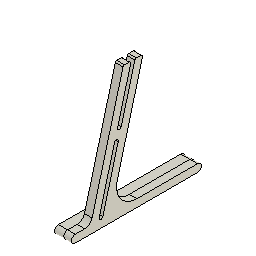
LCA 2021 Badge Stand v3 (Autodesk Fusion 360 design; units mm, degrees)
Autodesk Fusion 360 part; units mm, degrees
note: some values were not read from the file. Set by a fixed rule: which sketch regions a step uses.
sketch "Sketch1" plane through (0, 0, 0) normal (1, 0, 0) x (0, 1, 0)
  circle A0 centre (-67.0553, 26.6271) radius 2.5
  line L0 (-67.0553, 29.1271) -> (12.9447, 29.1271)
  line L1 (12.9447, 29.1271) -> (12.9447, 24.1271)
  line L2 (12.9447, 24.1271) -> (-67.0553, 24.1271)
  line L3 (-67.0553, 24.1271) -> (-67.0553, 29.1271)
  circle A1 centre (12.9447, 26.6271) radius 2.5
  line L4 (-57.0553, 29.1271) -> (-57.0553, 44.2726) construction
  line L5 (-57.0553, 29.1271) -> (-35.818, 108.3859)
  line L6 (-34.8521, 109.1271) -> (-31.7462, 109.1271)
  line L7 (-30.7803, 107.8682) -> (-51.8789, 29.1271)
  line L8 (-49.2908, 29.1271) -> (-28.0534, 108.3859)
  line L9 (-23.0157, 107.8682) -> (-44.1144, 29.1271)
  line L10 (-27.0875, 109.1271) -> (-23.9817, 109.1271)
  arc A2 (-34.8521, 109.1271) -> (-35.818, 108.3859) centre (-34.8521, 108.1271) ccw
  arc A3 (-30.7803, 107.8682) -> (-31.7462, 109.1271) centre (-31.7462, 108.1271) ccw
  arc A4 (-27.0875, 109.1271) -> (-28.0534, 108.3859) centre (-27.0875, 108.1271) ccw
  arc A5 (-23.0157, 107.8682) -> (-23.9817, 109.1271) centre (-23.9817, 108.1271) ccw
  line L11 (-37.233, 74.1271) -> (-39.8212, 74.1271)
  line L12 (-41.161, 69.1271) -> (-38.5728, 69.1271)
  circle A6 centre (-40.2305, 67.855) radius 1.272
  circle A7 centre (-38.1922, 75.3771) radius 1.25
  line L13 (-38.1922, 75.3771) -> (-39.4422, 75.3771)
  line L14 (-38.1922, 75.3771) -> (-36.9422, 75.3771)
  line L15 (-40.2305, 67.855) -> (-41.5025, 67.8524)
  line L16 (-40.2305, 67.855) -> (-38.9585, 67.8577)
  circle A8 centre (-50.2499, 30.3771) radius 1.25
  dimension "d6" = 5
  dimension "d7" = 80
  dimension "d8" = 5
  dimension "d9" = 10
  dimension "d10" = 2.5
  dimension "d11" = 5
  dimension "d12" = 5
  dimension "d13" = 75
  dimension "d16" = 1
  dimension "d17" = 1
  dimension "d18" = 1
  dimension "d19" = 1
  dimension "d20" = 80
  dimension "d35" = 5
  dimension "d36" = 35
  constraint horizontal L0
  constraint vertical L1
  constraint horizontal L2
  constraint vertical L3
  constraint coincident A0.centre L3
  constraint tangent A0 L0
  constraint tangent A0 L2
  constraint midpoint L1 A1.centre
  constraint coincident L0 L4.start
  constraint perpendicular L0 L4
  constraint perpendicular L4 L6
  constraint parallel L5 L7
  constraint coincident L0 L7.end
  constraint parallel L8 L9
  constraint coincident L0 L8.start
  constraint coincident L0 L9.end
  constraint collinear L6 L10
  constraint tangent L5 A2
  constraint tangent L6 A2
  constraint tangent L6 A3
  constraint tangent L7 A3
  constraint tangent L8 A4
  constraint tangent L10 A4
  constraint tangent L9 A5
  constraint tangent L10 A5
  constraint coincident L8 L11.start
  constraint coincident L7 L11.end
  constraint horizontal L11
  constraint coincident L7 L12.start
  constraint coincident L8 L12.end
  constraint parallel L11 L12
  constraint tangent L12 A6
  constraint tangent L8 A6
  constraint tangent L11 A7
  constraint tangent L7 A7
  constraint tangent L8 A7
  constraint coincident A7.centre L13.start
  constraint coincident A7 L13.end
  constraint horizontal L13
  constraint coincident A7 L14.end
  constraint parallel L13 L14
  constraint coincident A6.centre L15.start
  constraint coincident A6 L15.end
  constraint coincident L7 L15.end
  constraint coincident A6 L16.end
  constraint parallel L15 L16
  constraint tangent L0 A8
  constraint tangent L7 A8
  constraint tangent L8 A8
  measures "d6" diameter of A0
  measures "d7" distance of L0.start L1
  measures "d8" diameter of A1
  measures "d9" distance of L0.start L4
  measures "d10" distance of L7 L8
  measures "d11" distance of L5 L7
  measures "d12" distance of L8 L9
  measures "d13" angle of L0 L7
  measures "d16" radius of A2
  measures "d17" radius of A3
  measures "d18" radius of A4
  measures "d19" radius of A5
  measures "d20" distance of L0 L6
  measures "d35" distance of L11 L12
  measures "d36" distance of L6 L11
extrude "Extrude1" add sketch "Sketch1" along normal blind 5 contours A0 L3 | A0 L0 L2 A1 | A0 L3 | L0 L5 L6 L7 A2 A3 A6 | L1 A1 | L1 A1 | L0 L7 A8 | L0 L8 A8 | L0 L8 L9 L10 A4 A5 | L7 A6 | L8 L12 A6 | L7 L12 A6 | L7 L8 L11 L12 | L7 L11 A7 | L8 L11 A7 makes body 1
fillet "FrontFillet" radius 5 1 edges at (2.5, -57.0553, 29.1271) on bodies 1
fillet "RearArmFillet" radius 13.3333 1 edges at (2.5, -44.1144, 29.1271) on bodies 1
extrude "AddBaseThickener" add sketch "Sketch1" against normal blind 6 separate body contours A0 L3 | A0 L0 L2 A1 | A0 L3 | L1 A1 | L1 A1 makes body 2
copy_body "CutPasteBodies2" bodies 1 2 removing the originals makes body 3 makes body 4 in component "Component"
component "Component" placed x (1, 0, 0) y (0, 1, 0) z (0, 0, 1) at (0, 0, 0)
equation "boardthickness = 2.5 mm"
equation "fillet = 1 mm"
equation "basethickness = 5 mm"
equation "baselength = 80 mm"
equation "base_setback = 10 mm"
equation "d6 = basethickness"
equation "d7 = baselength"
equation "d8 = d6"
equation "d9 = base_setback"
equation "d10 = boardthickness"
equation "d11 = basethickness"
equation "d12 = d11"
equation "d13 = board_angle"
equation "board_angle = 75 deg"
equation "d16 = fillet"
equation "d17 = fillet"
equation "d20 = holderheight"
equation "holderheight = 80 mm"
equation "d25 = basethickness"
equation "d27 = holderheight / 6"
equation "d28 = -thickener"
equation "thickener = 6 mm"
equation "d35 = basethickness"
equation "d36 = topBadgeSpace"
equation "topBadgeSpace = 35 mm" comment "The depth of the \"slots\" for the holder"
named bodies: "MainBit", "Thicker_Base"
